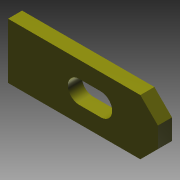
# Autodesk Inventor part: UB16NKG015F-NR
Saved by Autodesk Inventor 2015 SP1 (Build 190203100, 203)
## iProperties
Category: Electrical
Company: Autodesk Inc.
Created: 2014-12-16
Part Number: UB16NKG015F-NR
Catalog Web Link: http://www.nkkswitches.com/
Description: UB_ill_solder lug-Illuminated Pushbuttons - Series UB
Vendor: NKK Switches
Document SubType Name: Modeling
Designer: Autodesk Inc.
Manufacturer: NKKSWITCHES
Mass: 0.00472135 g
Surface Area: 0.278427 cm^2
Volume: 0.00472135 cm^3
Density: 1 g/cm^3
Material: Generic
Appearance: PSOLRGB-255-255-0
PSOL_IDENT_2: 07:10:00},{VERSION=},{LINEID=10},{LINESUBID=-1},{WBVAR=CR}  {NB=UBG-solder lug},{LINA=UBG-solder lug
PSOL_IDENT_3: },{KT=DUMMY},{SRS=UB},{COL=1.00,1.00,0.00,0.00},{CR=G}
SUPPLIER: NKKSWITCHES
Title: UBG-solder lug
Author: Autodesk Inc.
Comments: Illuminated Pushbuttons - Series UB
Autodesk Inventor part; units mm, degrees
sketch "Sketch_1" plane through (0, 0, 0) normal (0, 0, 1) x (1, 0, 0)
  line L0 (0, 1.0033) -> (0, -1.0033)
  line L1 (0, -1.0033) -> (4.7752, -1.0033)
  line L2 (4.7752, -1.0033) -> (5.4102, -0.3683)
  line L3 (5.4102, -0.3683) -> (5.4102, 0.3683)
  line L4 (5.4102, 0.3683) -> (4.7752, 1.0033)
  line L5 (4.7752, 1.0033) -> (0, 1.0033)
  arc A0 (2.5654, 0.4064) -> (2.5654, -0.4064) centre (2.5654, 0) ccw
  line L6 (2.5654, -0.4064) -> (3.3528, -0.4064)
  arc A1 (3.3528, -0.4064) -> (3.3528, 0.4064) centre (3.3528, 0) ccw
  line L7 (3.3528, 0.4064) -> (2.5654, 0.4064)
  constraints: 16 end point, 4 point on circle, 2 centre point
extrude "Extrusion1" add sketch "Sketch_1" along normal mid plane 0.508
ref_plane "P_XY" through (0, 0, 0) normal (1, 0, 0) x (0, 0, -1)
ref_plane "P_YZ" through (0, 0, 0) normal (0, 0, -1) x (0, 1, 0)
ref_plane "P_ZX" through (0, 0, 0) normal (0, 1, 0) x (1, 0, 0)
body "Solid1"
